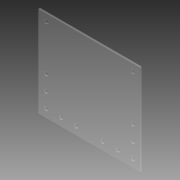
# Autodesk Inventor part: bambar plate
Saved by Autodesk Inventor 2011 SP1 (Build 150282100, 282)
## iProperties
Created: 2012-01-20
Part Number: bambar plate
Document SubType Name: Modeling
Designer: Christopher
Density: 1 g/cm^3
Author: Christopher
Autodesk Inventor part; units mm, degrees
ref_plane "YZ Plane" through (0, 0, 0) normal (1, 0, 0) x (0, 1, 0)
ref_plane "XZ Plane" through (0, 0, 0) normal (0, 1, 0) x (-1, 0, 0)
ref_plane "XY Plane" through (0, 0, 0) normal (0, 0, 1) x (1, 0, 0)
sketch "Sketch1" plane through (0, 0, 0) normal (0, 0, 1) x (1, 0, 0)
  line L0 (0, 0) -> (171.45, 0)
  line L1 (171.45, 0) -> (171.45, 152.4)
  line L2 (171.45, 152.4) -> (0, 152.4)
  line L3 (0, 152.4) -> (0, 0)
  point P0 (12.7, 12.7)
  point P1 (12.7, 38.1)
  point P2 (12.7, 63.5)
  point P3 (38.1, 12.7)
  point P4 (63.5, 12.7)
  point P5 (107.95, 12.7)
  point P6 (133.35, 12.7)
  point P7 (158.75, 12.7)
  point P8 (158.75, 38.1)
  point P9 (158.75, 63.5)
  point P10 (158.75, 139.7)
  point P11 (12.7, 139.7)
  dimension "d0" = 171.45
  dimension "d1" = 152.4
  dimension "d2" = 12.7
  dimension "d3" = 12.7
  dimension "d4" = 12.7
  dimension "d5" = 25.4
  dimension "d6" = 25.4
  dimension "d7" = 25.4
  dimension "d8" = 25.4
  dimension "d9" = 25.4
  dimension "d10" = 25.4
  dimension "d11" = 25.4
  dimension "d12" = 25.4
  dimension "d22" = 12.7
  constraints: 8 end point, 6 horizontal alignment, 6 vertical alignment, 2 parallel, 1 horizontal, 1 perpendicular
  measures "d0" distance of L1.end L2.end
  measures "d1" distance of L2.end L0.start
  measures "d2" distance from line of L0 point (63.5, 12.7)
  measures "d3" distance from line of L3 point (12.7, 38.1)
  measures "d4" distance from line of L1 point (158.75, 38.1)
  measures "d5" distance of point (158.75, 12.7) point (133.35, 12.7)
  measures "d6" distance of point (107.95, 12.7) point (133.35, 12.7)
  measures "d7" distance of point (158.75, 12.7) point (158.75, 38.1)
  measures "d8" distance of point (158.75, 38.1) point (158.75, 63.5)
  measures "d9" distance of point (12.7, 12.7) point (38.1, 12.7)
  measures "d10" distance of point (38.1, 12.7) point (63.5, 12.7)
  measures "d11" distance of point (12.7, 38.1) point (12.7, 12.7)
  measures "d12" distance of point (12.7, 38.1) point (12.7, 63.5)
  measures "d22" distance from line of L2 point (12.7, 139.7)
extrude "Extrusion1" add sketch "Sketch1" against normal blind 3.175
hole "Hole1" at (12.7, 12.7, 0) at (12.7, 38.1, 0) at (12.7, 63.5, 0) at (38.1, 12.7, 0) at (63.5, 12.7, 0) at (107.95, 12.7, 0) at (133.35, 12.7, 0) at (158.75, 12.7, 0) at (158.75, 38.1, 0) at (158.75, 63.5, 0) at (12.7, 139.7, 0) at (158.75, 139.7, 0) direction (0, 0, -1) diameter 6.35 depth 25.4 tip angle 118
body "Solid1"
